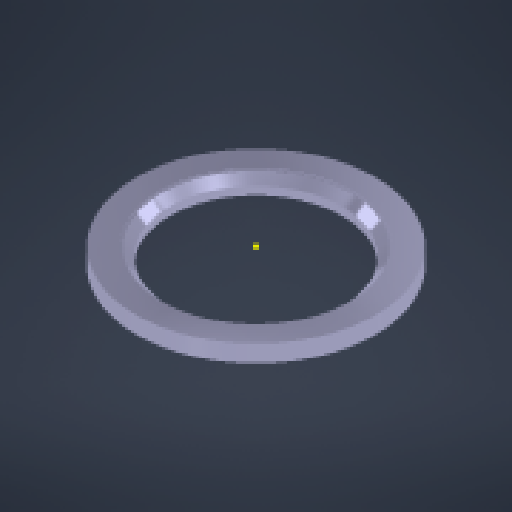
# Autodesk Inventor part: CR_OUTSIDE,BOTTOM,REV-ENG
Saved by Autodesk Inventor 2026.2 (Build 302298010, 298A)
## iProperties
Created: 2026-03-05
Part Number: CR_OUTSIDE,BOTTOM,REV-ENG
Material: Stainless Steel, 316L
Document SubType Name: Modeling
Designer: 4aida
Density: 8 g/cm^3
Appearance: Blue Chrome
Author: 4aida
Autodesk Inventor part; units mm, degrees
ref_plane "YZ Plane" through (0, 0, 0) normal (1, 0, 0) x (0, 1, 0)
ref_plane "XZ Plane" through (0, 0, 0) normal (0, 1, 0) x (-1, 0, 0)
ref_plane "XY Plane" through (0, 0, 0) normal (0, 0, 1) x (1, 0, 0)
sketch "Sketch1" plane through (0, 0, 0) normal (1, 0, 0) x (0, 1, 0)
  line L0 (-4.2955, 0) -> (4.2955, 0)
  line L1 (0, 35) -> (0, 28.0784)
  line L2 (-2.5784, 25.25) -> (-5, 25.25)
  line L3 (-5, 25.25) -> (-5, 35)
  line L4 (-5, 35) -> (0, 35)
  line L5 (-2.5784, 25.25) -> (-0.25, 27.5784)
  line L6 (-0.25, 27.5784) -> (-0.25, 28.0784)
  line L7 (-0.25, 28.0784) -> (0, 28.0784)
  line L8 (0, 22.1716) -> (-2.8284, 25) construction
  line L9 (-2.8284, 25) -> (0, 27.8284) construction
  line L10 (0, 27.8284) -> (2.8284, 25) construction
  line L11 (2.8284, 25) -> (0, 22.1716) construction
  line L12 (0, 22.1716) -> (0, 27.8284) construction
  line L13 (-2.8284, 25) -> (2.8284, 25) construction
  point P0 (0, 0)
  point P1 (0, 0)
  point P2 (0, 25)
  point P3 (-1.4142, 26.4142)
  dimension "d1" = 5
  dimension "d2" = 0.5
  dimension "d3" = 0.25
  dimension "d4" = 135
  dimension "d7" = 4
  dimension "d8" = 50
  dimension "d9" = 0.25
  dimension "d10" = 70
  constraints: 28 end point, 6 perpendicular, 5 midpoint, 2 parallel, 2 vertical, 1 coincident, 1 collinear, 1 horizontal, 1 point on line, 1 vertical alignment
  measures "d1" distance between parallel lines of L3 L1
  measures "d2" distance of L5.end L6.end
  measures "d3" distance of L6.end L1.end
  measures "d4" angle of L2 L5
  measures "d7" distance of L9.end L10.end
  measures "d8" diameter of L10.end L0
  measures "d9" distance from line of L8.end L2
  measures "d10" diameter of L4 L0
revolve "Revolution1" add sketch "Sketch1" angle 360 about axis through (0, -4.2955, 0) along (0, 1, 0)
sketch "Sketch2" plane through (0, 0, 0) normal (0, 1, 0) x (1, 0, 0)
  point P0 (0, 0)
sketch "Sketch3" plane through (0, -5, 0) normal (0, -1, 0) x (1, 0, 0)
  circle A0 centre (0, 0) radius 35
  arc A1 (2.5275, 28.8896) -> (-2.5275, 28.8896) centre (0, 0) ccw construction
  arc A2 (2.2508, 25.7267) -> (-2.2508, 25.7267) centre (0, 0) ccw
  arc A3 (2.2508, 25.7267) -> (5.3051, 27.3516) centre (2.5275, 28.8896) ccw
  arc A4 (-5.3051, 27.3516) -> (-2.2508, 25.7267) centre (-2.5275, 28.8896) ccw
  line L0 (2.5275, 28.8896) -> (0, 0) construction
  line L1 (0, 0) -> (-2.5275, 28.8896) construction
  arc A5 (7.0816, 28.1221) -> (5.3051, 27.3516) centre (6.6939, 26.5826) ccw
  arc A6 (-5.3051, 27.3516) -> (-7.0816, 28.1221) centre (-6.6939, 26.5826) ccw
  arc A7 (-25.7267, 2.2508) -> (-27.3516, 5.3051) centre (-28.8896, 2.5275) ccw
  arc A8 (-28.1221, 7.0816) -> (-27.3516, 5.3051) centre (-26.5826, 6.6939) ccw
  arc A9 (-27.3516, -5.3051) -> (-28.1221, -7.0816) centre (-26.5826, -6.6939) ccw
  arc A10 (-27.3516, -5.3051) -> (-25.7267, -2.2508) centre (-28.8896, -2.5275) ccw
  arc A11 (-25.7267, 2.2508) -> (-25.7267, -2.2508) centre (0, 0) ccw
  arc A12 (-2.2508, -25.7267) -> (-5.3051, -27.3516) centre (-2.5275, -28.8896) ccw
  arc A13 (-7.0816, -28.1221) -> (-5.3051, -27.3516) centre (-6.6939, -26.5826) ccw
  arc A14 (5.3051, -27.3516) -> (7.0816, -28.1221) centre (6.6939, -26.5826) ccw
  arc A15 (5.3051, -27.3516) -> (2.2508, -25.7267) centre (2.5275, -28.8896) ccw
  arc A16 (-2.2508, -25.7267) -> (2.2508, -25.7267) centre (0, 0) ccw
  arc A17 (25.7267, -2.2508) -> (27.3516, -5.3051) centre (28.8896, -2.5275) ccw
  arc A18 (28.1221, -7.0816) -> (27.3516, -5.3051) centre (26.5826, -6.6939) ccw
  arc A19 (27.3516, 5.3051) -> (28.1221, 7.0816) centre (26.5826, 6.6939) ccw
  arc A20 (27.3516, 5.3051) -> (25.7267, 2.2508) centre (28.8896, 2.5275) ccw
  arc A21 (25.7267, -2.2508) -> (25.7267, 2.2508) centre (0, 0) ccw
  arc A22 (-7.0816, 28.1221) -> (-28.1221, 7.0816) centre (0, 0) ccw
  arc A23 (-28.1221, -7.0816) -> (-7.0816, -28.1221) centre (0, 0) ccw
  arc A24 (7.0816, -28.1221) -> (28.1221, -7.0816) centre (0, 0) ccw
  arc A25 (28.1221, 7.0816) -> (7.0816, 28.1221) centre (0, 0) ccw
  point P0 (0, 29)
  dimension "d13" = 70
  dimension "d16" = 10
  dimension "d17" = 3.175
  dimension "d18" = 1.5875
  dimension "d21" = 360
  dimension "d23" = 29
  constraints: 52 point on circle, 26 centre point, 6 tangent, 4 end point, 2 coincident, 1 concentric, 1 equal radius, 1 vertical alignment, 65 other
  measures "d13" diameter of A0
  measures "d16" angle of L1 L0
  measures "d17" radius of A3
  measures "d18" radius of A5
  measures "d23" radius of A25
extrude "Extrusion1" add sketch "Sketch3" along normal blind 1.5
body "Solid1"
